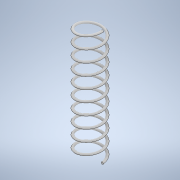
# Autodesk Inventor part: spring
Saved by Autodesk Inventor 2021 (Build 250183000, 183)
## iProperties
Created: 2021-02-21
Part Number: spring
Material: Generic
Document SubType Name: Modeling
Designer: Dell
Density: 1 g/cm^3
Appearance: Default
Author: Dell
Autodesk Inventor part; units mm, degrees
ref_plane "YZ Plane" through (0, 0, 0) normal (1, 0, 0) x (0, 1, 0)
ref_plane "XZ Plane" through (0, 0, 0) normal (0, 1, 0) x (-1, 0, 0)
ref_plane "XY Plane" through (0, 0, 0) normal (0, 0, 1) x (1, 0, 0)
sketch "Sketch1" plane through (0, 0, 0) normal (0, 0, 1) x (1, 0, 0)
  line L0 (0, 0) -> (0, 0.1)
  line L1 (0, 0) -> (0.108, 0)
  circle A0 centre (0.108, 0) radius 0.01
  dimension "d0" = 0.1
  dimension "d1" = 0.108
  dimension "d2" = 0.02
  constraints: 4 end point, 1 centre point, 1 coincident, 1 horizontal, 1 vertical
  measures "d0" distance of L0.start L0.end
  measures "d1" distance of L0.start L1.end
  measures "d2" diameter of A0
coil "Coil1" sketch "Sketch1" operation add axis through (0, 0, 0) along (0, 1, 0) pitch 0.1 turns 10 hand right
body "Solid1"
